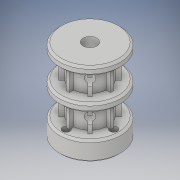
# Autodesk Inventor part: КВ33.044.302 - Шкив
Saved by Autodesk Inventor 2019 (Build 230136000, 136)
## iProperties
Created: 2019-07-23
Part Number: КВ33.044.302 - Шкив
Material: Типовые
Document SubType Name: Modeling
Designer: user
Density: 1 g/cm^3
Appearance: По умолчанию
Author: user
Autodesk Inventor part; units mm, degrees
ref_plane "YZ Plane" through (0, 0, 0) normal (1, 0, 0) x (0, 1, 0)
ref_plane "XZ Plane" through (0, 0, 0) normal (0, 1, 0) x (-1, 0, 0)
ref_plane "XY Plane" through (0, 0, 0) normal (0, 0, 1) x (1, 0, 0)
sketch "Эскиз1" plane through (0, 0, 0) normal (0, 1, 0) x (-1, 0, 0)
  circle A0 centre (0, 0) radius 11
  circle A1 centre (0, 8.58) radius 1.35
  circle A2 centre (-8.58, 0) radius 1.35
  circle A3 centre (0, -8.58) radius 1.35
  circle A4 centre (8.58, 0) radius 1.35
  circle A5 centre (0, 0) radius 2.5
  dimension "d0" = 22
  dimension "d1" = 2.7
  dimension "d2" = 8.58
  dimension "d5" = 360
  dimension "d7" = 5
  constraints: 6 centre point, 2 coincident, 9 other
  measures "d0" diameter of A0
  measures "d1" diameter of A1
  measures "d2" distance of A0.centre A1.centre
  measures "d7" diameter of A5
extrude "Выдавливание1" add sketch "Эскиз1" along normal blind 7
sketch "Эскиз2" plane through (0, 7, 0) normal (0, 1, 0) x (1, 0, 0)
  circle A0 centre (0, 0) radius 6.5
  dimension "d10" = 13
  constraints: 1 centre point, 1 coincident
  measures "d10" diameter of A0
extrude "Выдавливание2" add sketch "Эскиз2" along normal blind 8.5
sketch "Эскиз3" plane through (0, 15.5, 0) normal (0, 1, 0) x (1, 0, 0)
  circle A0 centre (0, 0) radius 11
  constraints: 1 centre point, 1 coincident
extrude "Выдавливание3" add sketch "Эскиз3" along normal blind 3
sketch "Эскиз4" plane through (0, 18.5, 0) normal (0, 1, 0) x (1, 0, 0)
  circle A0 centre (0, 0) radius 6.5
  dimension "d15" = 13
  constraints: 1 centre point, 1 coincident
  measures "d15" diameter of A0
extrude "Выдавливание4" add sketch "Эскиз4" along normal blind 8.5
sketch "Эскиз5" plane through (0, 27, 0) normal (0, 1, 0) x (1, 0, 0)
  circle A0 centre (0, 0) radius 11
  dimension "d18" = 22
  constraints: 1 centre point, 1 coincident
  measures "d18" diameter of A0
extrude "Выдавливание5" add sketch "Эскиз5" along normal blind 3
chamfer "Фаска1" distance 0.75 angle 45 6 edges at (-11, 30, 0) (-11, 18.5, 0) (-11, 15.5, 0) (-11, 27, 0) (11, 0, 0) (11, 7, 0)
sketch "Эскиз6" plane through (0, 30, 0) normal (0, 1, 0) x (1, 0, 0)
  line L0 (0.5734, -8.0304) -> (-0.5736, -8.0304)
  line L1 (-0.5736, -8.0304) -> (-0.5736, 8.0304)
  line L2 (-0.5736, 8.0304) -> (0.5734, 8.0304)
  line L3 (0.5734, 8.0304) -> (0.5734, -8.0304)
  line L4 (0.5734, -8.0304) -> (-0.5736, 8.0304) construction
  line L5 (-0.5736, -8.0304) -> (0.5734, 8.0304) construction
  line L6 (-8.0304, -0.5734) -> (-8.0304, 0.5736)
  line L7 (-8.0304, 0.5736) -> (8.0304, 0.5736)
  line L8 (8.0304, 0.5736) -> (8.0304, -0.5734)
  line L9 (8.0304, -0.5734) -> (-8.0304, -0.5734)
  line L10 (-8.0304, -0.5734) -> (8.0304, 0.5736) construction
  line L11 (-8.0304, 0.5736) -> (8.0304, -0.5734) construction
  line L12 (6.0838, -5.2729) -> (5.2728, -6.0839)
  line L13 (5.2728, -6.0839) -> (-6.0839, 5.2728)
  line L14 (-6.0839, 5.2728) -> (-5.2729, 6.0838)
  line L15 (-5.2729, 6.0838) -> (6.0838, -5.2729)
  line L16 (6.0838, -5.2729) -> (-6.0839, 5.2728) construction
  line L17 (5.2728, -6.0839) -> (-5.2729, 6.0838) construction
  line L18 (-5.2728, -6.0839) -> (-6.0838, -5.2729)
  line L19 (-6.0838, -5.2729) -> (5.2729, 6.0838)
  line L20 (5.2729, 6.0838) -> (6.0839, 5.2728)
  line L21 (6.0839, 5.2728) -> (-5.2728, -6.0839)
  line L22 (-5.2728, -6.0839) -> (5.2729, 6.0838) construction
  line L23 (-6.0838, -5.2729) -> (6.0839, 5.2728) construction
  point P0 (0, 0)
  dimension "d24" = 1.147
  dimension "d25" = 16.0608
  dimension "d26" = 1.147
  dimension "d27" = 16.0608
  dimension "d28" = 1.147
  dimension "d29" = 16.0608
  dimension "d30" = 1.147
  dimension "d31" = 16.0608
  constraints: 48 end point, 8 parallel, 4 perpendicular, 1 horizontal
  measures "d24" distance of L1.end L2.end
  measures "d25" distance of L0.end L1.end
  measures "d26" distance of L7.end L8.end
  measures "d27" distance of L6.end L7.end
  measures "d28" distance of L16.end L15.start
  measures "d29" distance of L13.start L16.end
  measures "d30" distance of L19.end L20.end
  measures "d31" distance of L18.end L19.end
extrude "Выдавливание6" add sketch "Эскиз6" against normal up to surface (23 mm away)
sketch "Эскиз7" plane through (5.2728, 7, 6.0839) normal (0.7071, 0, 0.7071) x (0.7071, 0, -0.7071)
  circle A0 centre (0.6, 16.1997) radius 1.5
  circle A1 centre (0.6, 4.25) radius 1.5
  point P0 (0.5736, -7)
  dimension "d37" = 3
  dimension "d38" = 3
  constraints: 2 centre point
  measures "d37" diameter of A0
  measures "d38" diameter of A1
extrude "Выдавливание7" cut sketch "Эскиз7" against normal through all
sketch "Эскиз8" plane through (0, 30, 0) normal (0, 1, 0) x (1, 0, 0)
  circle A0 centre (0, 0) radius 2.5
  dimension "d41" = 5
  constraints: 1 centre point, 1 coincident
  measures "d41" diameter of A0
extrude "Выдавливание8" cut sketch "Эскиз8" against normal through all
